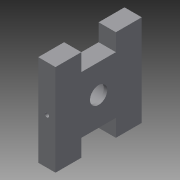
# Autodesk Inventor part: prepazka_kola
Saved by Autodesk Inventor 2015 (Build 190159000, 159)
## iProperties
Created: 2012-08-21
Part Number: prepazka_kola
Material: Generic
Document SubType Name: Modeling
Designer: idle-rug
Density: 1 g/cm^3
Appearance: Default
Author: idle-rug
Autodesk Inventor part; units mm, degrees
ref_plane "YZ Plane" through (0, 0, 0) normal (1, 0, 0) x (0, 1, 0)
ref_plane "XZ Plane" through (0, 0, 0) normal (0, 1, 0) x (-1, 0, 0)
ref_plane "XY Plane" through (0, 0, 0) normal (0, 0, 1) x (1, 0, 0)
sketch "Sketch3" plane through (0, 0, 0) normal (1, 0, 0) x (0, 1, 0)
  line L0 (25, -26.5) -> (-25, -26.5)
  line L1 (-25, -26.5) -> (-25, 26.5)
  line L2 (-25, 26.5) -> (25, 26.5)
  line L3 (25, 26.5) -> (25, -26.5)
  line L4 (25, -26.5) -> (-25, 26.5) construction
  line L5 (-25, -26.5) -> (25, 26.5) construction
  line L6 (25, 26.5) -> (10, 26.5)
  line L7 (10, 26.5) -> (10, 16.5)
  line L8 (10, 16.5) -> (-10, 16.5)
  line L9 (-10, 16.5) -> (-10, 26.5)
  line L10 (-10, 26.5) -> (-25, 26.5)
  line L11 (25, -26.5) -> (10, -26.5)
  line L12 (10, -26.5) -> (10, -16.5)
  line L13 (10, -16.5) -> (-10, -16.5)
  line L14 (-10, -16.5) -> (-10, -26.5)
  line L15 (-10, -26.5) -> (-25, -26.5)
  point P0 (0, 0)
  dimension "d0" = 50
  dimension "d1" = 53
  dimension "d2" = 15
  dimension "d3" = 10
  dimension "d4" = 20
  dimension "d5" = 10
  dimension "d6" = 15
  dimension "d7" = 10
  dimension "d8" = 20
  dimension "d9" = 10
  dimension "d10" = 15
  constraints: 32 end point, 4 parallel, 4 point on line, 3 perpendicular, 2 midpoint, 1 collinear, 1 horizontal
  measures "d0" distance of L1.end L2.end
  measures "d1" distance of L0.end L1.end
  measures "d2" distance of L2.end L6.end
  measures "d3" distance of L6.end L7.end
  measures "d4" distance of L7.end L8.end
  measures "d5" distance of L8.end L9.end
  measures "d6" distance of L0.start L11.end
  measures "d7" distance of L11.end L12.end
  measures "d8" distance of L12.end L13.end
  measures "d9" distance of L13.end L14.end
  measures "d10" distance of L14.end L0.end
extrude "Extrusion1" add sketch "Sketch3" along normal blind 10 contours L0 L12 L13 L14 L1 L2 L9 L8 L7 L3
sketch "Sketch5" plane through (10, 0, 0) normal (1, 0, 0) x (0, 0, -1)
  circle A0 centre (0, 0) radius 7.5
  circle A1 centre (0, 0) radius 5
  dimension "d13" = 15
  dimension "d33" = 10
  constraints: 2 centre point, 2 coincident
  measures "d13" diameter of A0
  measures "d33" diameter of A1
sketch "Sketch6" plane through (0, -25, -26.5) normal (0, -1, 0) x (1, 0, 0)
  circle A0 centre (5, 26.5) radius 1.25
  dimension "d30" = 2.5
  constraints: 1 centre point
  measures "d30" diameter of A0
extrude "Extrusion2" cut sketch "Sketch5" against normal blind 10 contours A0 | A1
extrude "Extrusion3" cut sketch "Sketch6" against normal blind 10
extrude "Extrusion4" add sketch "Sketch5" against normal blind 2
fillet "Fillet1" radius 2 1 edges at (0, 0, 7.5)
body "Solid1"
